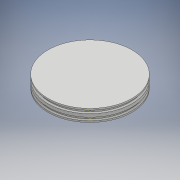
# Autodesk Inventor part: PulleyAdapter
Saved by Autodesk Inventor 2017 (Build 210142000, 142)
## iProperties
Created: 2017-02-11
Part Number: PulleyAdapter
Material: Generic
Document SubType Name: Modeling
Designer: aribu
Density: 1 g/cm^3
Appearance: Default
Author: aribu
Autodesk Inventor part; units mm, degrees
ref_plane "YZ Plane" through (0, 0, 0) normal (1, 0, 0) x (0, 1, 0)
ref_plane "XZ Plane" through (0, 0, 0) normal (0, 1, 0) x (-1, 0, 0)
ref_plane "XY Plane" through (0, 0, 0) normal (0, 0, 1) x (1, 0, 0)
sketch "Sketch3" plane through (0, 0, 0) normal (0, 0, 1) x (1, 0, 0)
  circle A0 centre (0, 0) radius 4.45
  dimension "d11" = 8.9
  constraints: 1 centre point, 1 coincident
  measures "d11" diameter of A0
extrude "Extrusion3" add sketch "Sketch3" along normal blind 10
sketch "Sketch4" plane through (0, 0, 10) normal (0, 0, 1) x (1, 0, 0)
  circle A0 centre (0, 0) radius 27.5
  dimension "d14" = 55
  constraints: 1 centre point, 1 coincident
  measures "d14" diameter of A0
extrude "Extrusion4" add sketch "Sketch4" along normal blind 8
ref_plane "Work Plane2" through (0, 0, 12) normal (0, 0, 1) x (1, 0, 0)
ref_plane "Work Plane1" through (0, 0, 14) normal (0, 0, 1) x (1, 0, 0)
sketch "Sketch5" plane through (0, 0, 12) normal (0, 0, 1) x (1, 0, 0)
  circle A0 centre (0, 0) radius 26
  circle A1 centre (0, 0) radius 27.5
  dimension "d17" = 52
  dimension "d18" = 55
  constraints: 2 centre point, 2 coincident
  measures "d17" diameter of A0
  measures "d18" diameter of A1
extrude "Extrusion5" cut sketch "Sketch5" along normal mid plane 2
mirror "Mirror1" about plane through (0, 0, 14) normal (0, 0, 1) of "Extrusion5"
sketch "Sketch6" plane through (0, 0, 0) normal (0, 0, -1) x (-1, 0, 0)
  line L0 (2, 3) -> (-2, 3)
  line L1 (-2, 3) -> (-2, -3)
  line L2 (-2, -3) -> (2, -3)
  line L3 (2, -3) -> (2, 3)
  point P0 (0, 0)
  dimension "d21" = 6
  dimension "d22" = 4
  dimension "d23" = 3
  dimension "d24" = 2
  constraints: 8 end point, 2 parallel, 1 horizontal, 1 perpendicular
  measures "d21" distance of L2.end L0.start
  measures "d22" distance of L1.end L2.end
  measures "d23" distance from line of L2 point (0, 0)
  measures "d24" distance from line of L3 point (0, 0)
extrude "Extrusion6" cut sketch "Sketch6" against normal blind 10
ref_plane "Work Plane3" through (0, 0, 14) normal (0, 0, 1) x (1, 0, 0)
ref_plane "Work Plane4" through (0, 0, 16) normal (0, 0, 1) x (1, 0, 0)
equation "\"d23\" = 0.5 * d21"
equation "\"d24\" = 0.5 * d22"
body "Solid2"
